Autodesk Fusion 360 part; units mm, degrees
(part 13 of 13)
  line L672 (11.58, -20) -> (12.58, -20)
  line L673 (12.58, -20) -> (12.58, -21)
  line L674 (12.58, -21) -> (11.58, -21)
  line L675 (11.58, -21) -> (11.58, -20)
  line L676 (14.25, -20) -> (15.25, -20)
  line L677 (15.25, -20) -> (15.25, -21)
  line L678 (15.25, -21) -> (14.25, -21)
  line L679 (14.25, -21) -> (14.25, -20)
  line L680 (1.75, -16) -> (-1.75, -16)
  line L681 (-1.75, -16) -> (-1.75, 16)
  line L682 (-1.75, 16) -> (1.75, 16)
  line L683 (1.75, 16) -> (1.75, -16)
  line L684 (-17.25, 23) -> (-17.25, -23)
  line L685 (-17.25, -23) -> (17.25, -23)
  line L686 (17.25, -23) -> (17.25, 23)
  line L687 (17.25, 23) -> (-17.25, 23)
  circle A0 centre (0, -19) radius 1.5
  circle A1 centre (0, 19) radius 1.4142
  dimension "d29" = 2.8284
  dimension "d30" = 3
  measures "d29" diameter of A1
  measures "d30" diameter of A0
extrude "Extrude5" cut sketch "Sketch5" against normal blind 2 contours A0 | A1
sketch "Sketch6" plane through (0, -23, 0) normal (0, -1, 0) x (1, 0, 0)
  line L0 (-17.25, 0) -> (17.25, 0)
  line L1 (17.25, 0) -> (17.25, 8.5)
  line L2 (17.25, 8.5) -> (-17.25, 8.5)
  line L3 (-17.25, 8.5) -> (-17.25, 0)
  line L4 (-2, 5) -> (2, 5)
  line L5 (2, 5) -> (2, -5)
  line L6 (2, -5) -> (-2, -5)
  line L7 (-2, -5) -> (-2, 5)
  line L8 (-2, 5) -> (2, -5) construction
  line L9 (2, 5) -> (-2, -5) construction
  dimension "d33" = 10
  dimension "d34" = 4
  constraint horizontal L4
  constraint perpendicular L4 L5
  constraint parallel L4 L6
  constraint parallel L5 L7
  constraint coincident L8 origin
  constraint coincident L9 origin
  measures "d33" distance of L4.end L5.end
  measures "d34" distance of L4.start L4.end
extrude "Extrude6" add sketch "Sketch6" along normal blind 1 contours L0 L4 L5 L7
extrude "Extrude7" add 1 faces at (-0.6667, -24, 3.3333) along direction (0, 1, 0) blind 48
extrude "Extrude8" cut 1 faces at (-0.6667, 24, 3.3333) along direction (0, -1, 0) blind 2
sketch "Sketch7" plane through (17.25, 0, 0) normal (1, 0, 0) x (0, 1, 0)
  line L0 (-23, 0) -> (23, 0)
  line L1 (23, 0) -> (23, 8.5)
  line L2 (23, 8.5) -> (-23, 8.5)
  line L3 (-23, 8.5) -> (-23, 0)
  line L4 (-2, 0) -> (2, 0)
  line L5 (2, 0) -> (2, 5)
  line L6 (2, 5) -> (-2, 5)
  line L7 (-2, 5) -> (-2, 0)
  constraint horizontal L4
  constraint vertical L5
  constraint horizontal L6
  constraint vertical L7
  constraint coincident L0 L4.start
extrude "Extrude9" add sketch "Sketch7" along normal blind 1 contours L0 L4 L5 L6 L7
extrude "Extrude10" add 1 faces at (18.25, -0.6667, 3.3333) along direction (-1, 0, 0) blind 36.5
extrude "Extrude11" cut 1 faces at (-18.25, -0.6667, 3.3333) along direction (1, 0, 0) blind 2
